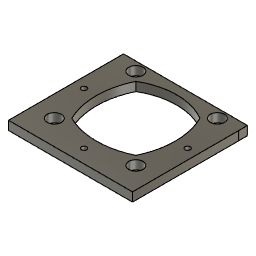
Ball bearing Spport for Steel Tube (Autodesk Fusion 360 design; units mm, degrees)
Autodesk Fusion 360 part; units mm, degrees
note: some values were not read from the file. Set by a fixed rule: which sketch regions a step uses.
sketch "Sketch1" plane through (0, 0, 0) normal (0, 0, 1) x (1, 0, 0)
  circle A0 centre (0, 0) radius 21.3
  line L0 (0, 0) -> (-15.0614, -15.0614)
  line L1 (0, 0) -> (21.3, 0) construction
  line L2 (-15.0614, -15.0614) -> (-23.0517, -23.0517)
  circle A1 centre (-23.0517, -23.0517) radius 11
  line L3 (0, 0) -> (15.0614, -15.0614)
  line L4 (15.0614, -15.0614) -> (23.0517, -23.0517)
  circle A2 centre (23.0517, -23.0517) radius 11
  circle A3 centre (-23.0517, 23.0517) radius 11
  circle A4 centre (23.0517, 23.0517) radius 11
  line L5 (-23.0517, 23.0517) -> (-35.0517, 23.0517)
  line L6 (-35.0517, 23.0517) -> (-35.0517, -36.9483)
  line L7 (23.0517, 23.0517) -> (35.0517, 23.0517)
  line L8 (35.0517, 23.0517) -> (35.0517, -36.9483)
  line L9 (35.0517, -36.9483) -> (-35.0517, -36.9483)
  line L10 (-23.0517, 23.0517) -> (23.0517, 23.0517)
  circle A5 centre (-23.0517, 23.0517) radius 4
  circle A6 centre (23.0517, 23.0517) radius 4
  circle A7 centre (23.0517, -23.0517) radius 4
  circle A8 centre (-23.0517, -23.0517) radius 4
  line L11 (-35.0517, 23.0517) -> (-35.0517, 24)
  line L12 (-35.0517, 24) -> (-35.0517, 28.0517)
  line L13 (-35.0517, 28.0517) -> (35.0082, 28.0517)
  line L14 (35.0082, 28.0517) -> (35.0517, 23.0517)
  line L15 (-23.0517, -23.0517) -> (-18.1019, -18.1019)
  line L16 (-23.0517, 23.0517) -> (-18.1019, 18.1019)
  line L17 (23.0517, 23.0517) -> (18.1019, 18.1019)
  line L18 (23.0517, 23.0517) -> (30.0517, 23.0517) construction
  line L19 (23.0517, -23.0517) -> (18.1019, -18.1019)
  arc A9 (18.1019, 18.1019) -> (-18.1019, 18.1019) centre (0, -12.5239) ccw
  line L20 (0, 0) -> (-21.3, 0)
  line L21 (-21.3, 0) -> (-22.3, 0)
  arc A10 (-18.1019, 18.1019) -> (-18.1019, -18.1019) centre (18.8265, 0) ccw
  line L22 (0, 0) -> (0, 5) construction
  arc A11 (18.1019, -18.1019) -> (18.1019, 18.1019) centre (-18.8265, 0) ccw
  line L23 (0, 0) -> (0, -21.3)
  line L24 (0, -21.3) -> (0, -22.3)
  arc A12 (-18.1019, -18.1019) -> (18.1019, -18.1019) centre (0, 18.8265) ccw
  line L25 (0, 0) -> (0, -21.3)
  line L26 (0, -21.3) -> (0, -29.3)
  line L27 (-21.3, 0) -> (-29.3, 0)
  line L28 (21.3, 0) -> (29.3, 0)
  circle A13 centre (29.3, 0) radius 1.5
  circle A14 centre (0, -29.3) radius 1.5
  circle A15 centre (-29.3, 0) radius 1.5
  dimension "d1" = 42.6
  dimension "d2" = 135
  dimension "d3" = 11.3
  dimension "d4" = 22
  dimension "d5" = 11.3
  dimension "d6" = 22
  dimension "d7" = 12
  dimension "d8" = 60
  dimension "d9" = 12
  dimension "d10" = 60
  dimension "d11" = 8
  dimension "d12" = 8
  dimension "d13" = 8
  dimension "d14" = 8
  dimension "d15" = 5
  dimension "d16" = 7
  dimension "d17" = 7
  dimension "d18" = 135
  dimension "d19" = 7
  dimension "d20" = 7
  dimension "d25" = 1
  dimension "d26" = 1
  dimension "d27" = 8
  dimension "d28" = 8
  dimension "d29" = 8
  dimension "d30" = 3
  dimension "d31" = 3
  dimension "d32" = 3
  constraint coincident A0.centre L0.start
  constraint horizontal L1
  constraint coincident A0 L0.end
  constraint parallel L0 L2
  constraint coincident L2.end A1.centre
  constraint coincident A0 L3.end
  constraint perpendicular L0 L3
  constraint perpendicular L0 L4
  constraint coincident L4.end A2.centre
  constraint symmetric L1 A1 A3
  constraint symmetric L1 A2 A4
  constraint coincident A3.centre L5.start
  constraint horizontal L5
  constraint perpendicular L5 L6
  constraint coincident A4.centre L7.start
  constraint horizontal L7
  constraint perpendicular L7 L8
  constraint concentric A3 A5
  constraint concentric A4 A6
  constraint concentric A2 A7
  constraint concentric A1 A8
  constraint perpendicular L5 L11
  constraint perpendicular L5 L12
  constraint perpendicular L12 L13
  constraint parallel L2 L15
  constraint perpendicular L15 L16
  constraint horizontal L18
  constraint parallel L4 L19
  constraint coincident A0 L20.end
  constraint horizontal L20
  constraint parallel L20 L21
  constraint coincident L21.end A10
  constraint perpendicular L1 L22
  constraint symmetric L15.end L22 L19.end
  constraint symmetric L16.end L22 L17.end
  constraint symmetric A10 L22 A11
  constraint coincident A0 L23.end
  constraint perpendicular L1 L23
  constraint parallel L23 L24
  constraint coincident L24.end A12
  constraint parallel L24 L26
  constraint parallel L21 L27
  constraint perpendicular L8 L28
  constraint coincident L28.end A13.centre
  constraint coincident L26.end A14.centre
  constraint coincident L27.end A15.centre
  measures "d1" diameter of A0
  measures "d2" angle of L0 L1
  measures "d3" distance of L0.end L2.end
  measures "d4" diameter of A1
  measures "d5" distance of L3.end L4.end
  measures "d6" diameter of A2
  measures "d7" distance of A3.centre L5.end
  measures "d8" distance of L5.end L6.end
  measures "d9" distance of A4.centre L7.end
  measures "d10" distance of L7.end L8.end
  measures "d11" diameter of A5
  measures "d12" diameter of A6
  measures "d13" diameter of A7
  measures "d14" diameter of A8
  measures "d15" vertical distance of L7.end L13.end
  measures "d16" distance of L2.end L15.end
  measures "d17" distance of A3.centre L16.end
  measures "d18" angle of L17 L18
  measures "d19" distance of A4.centre L17.end
  measures "d20" distance of L4.end L19.end
  measures "d25" distance of L20.end L21.end
  measures "d26" distance of L23.end L24.end
  measures "d27" distance of L23.end L26.end
  measures "d28" distance of L20.end L27.end
  measures "d29" distance of L1.end L28.end
  measures "d30" diameter of A13
  measures "d31" diameter of A14
  measures "d32" diameter of A15
extrude "Extrude1" add sketch "Sketch1" along normal blind 5 contours A1 A2 A3 A4 L5 L6 L7 L8 L9 A10 A11 A12 | A2 A11 A12 | A4 L7 A6 L17 A11 | A3 L5 A5 L16 A10 | A1 A10 A12 | A4 L10 A9 | A4 L10 A6 L17 A9 | A4 L7 L10 A6 L13 | A4 L7 L13 L14 | A3 L5 L11 L12 L13 | A3 L5 L10 A5 L13 | A3 L10 A5 L16 A9 | A3 L10 A9 | A3 A4 L10 L13
